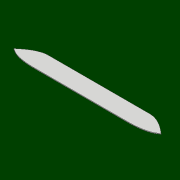
# Autodesk Inventor part: Part3
Saved by Autodesk Inventor 2018 (Build 220112000, 112)
## iProperties
Created: 2021-12-12
Part Number: Part3
Material: 一般
Document SubType Name: Modeling
Designer: gisen
Density: 1 g/cm^3
Appearance: 既定
Author: gisen
Autodesk Inventor part; units mm, degrees
ref_plane "YZ Plane" through (0, 0, 0) normal (1, 0, 0) x (0, 1, 0)
ref_plane "XZ Plane" through (0, 0, 0) normal (0, 1, 0) x (-1, 0, 0)
ref_plane "XY Plane" through (0, 0, 0) normal (0, 0, 1) x (1, 0, 0)
sketch "スケッチ1" plane through (0, 0, 0) normal (0, 0, 1) x (1, 0, 0)
  line L0 (357.9651, 235.4843) -> (362.63, 235.5738)
  line L1 (362.63, 235.5738) -> (367.0044, 235.8303)
  line L2 (367.0044, 235.8303) -> (371.0643, 236.2346)
  line L3 (371.0643, 236.2346) -> (374.8054, 236.7675)
  line L4 (374.8054, 236.7675) -> (378.2233, 237.4103)
  line L5 (378.2233, 237.4103) -> (381.3146, 238.1447)
  line L6 (381.3146, 238.1447) -> (384.0762, 238.953)
  line L7 (384.0762, 238.953) -> (386.507, 239.8191)
  line L8 (386.507, 239.8191) -> (388.6078, 240.7295)
  line L9 (388.6078, 240.7295) -> (390.3342, 241.6502)
  line L10 (390.3342, 241.6502) -> (395.2502, 244.5906)
  line L11 (395.2502, 244.5906) -> (390.8507, 248.2071)
  line L12 (390.8507, 248.2071) -> (388.6394, 249.9662)
  line L13 (388.6394, 249.9662) -> (386.4174, 251.6158)
  line L14 (386.4174, 251.6158) -> (384.2013, 253.1435)
  line L15 (384.2013, 253.1435) -> (381.995, 254.5468)
  line L16 (381.995, 254.5468) -> (379.8025, 255.8227)
  line L17 (379.8025, 255.8227) -> (377.6276, 256.9685)
  line L18 (377.6276, 256.9685) -> (375.4738, 257.9812)
  line L19 (375.4738, 257.9812) -> (373.3448, 258.8578)
  line L20 (373.3448, 258.8578) -> (371.2439, 259.5946)
  line L21 (371.2439, 259.5946) -> (369.1946, 260.1821)
  line L22 (369.1946, 260.1821) -> (368.499, 260.3499)
  line L23 (368.499, 260.3499) -> (367.8292, 260.4961)
  line L24 (367.8292, 260.4961) -> (367.1644, 260.6258)
  line L25 (367.1644, 260.6258) -> (366.5049, 260.7386)
  line L26 (366.5049, 260.7386) -> (365.8512, 260.8345)
  line L27 (365.8512, 260.8345) -> (365.2034, 260.9133)
  line L28 (365.2034, 260.9133) -> (364.5618, 260.9749)
  line L29 (364.5618, 260.9749) -> (363.9265, 261.0192)
  line L30 (363.9265, 261.0192) -> (363.298, 261.0459)
  line L31 (363.298, 261.0459) -> (362.6912, 261.0547)
  line L32 (362.6912, 261.0547) -> (216.4134, 261.0547)
  line L33 (216.4134, 261.0547) -> (215.8059, 261.0459)
  line L34 (215.8059, 261.0459) -> (215.1769, 261.0192)
  line L35 (215.1769, 261.0192) -> (214.5413, 260.9749)
  line L36 (214.5413, 260.9749) -> (213.8996, 260.9133)
  line L37 (213.8996, 260.9133) -> (213.2517, 260.8345)
  line L38 (213.2517, 260.8345) -> (212.598, 260.7385)
  line L39 (212.598, 260.7385) -> (211.9388, 260.6257)
  line L40 (211.9388, 260.6257) -> (211.2743, 260.4961)
  line L41 (211.2743, 260.4961) -> (210.6048, 260.3498)
  line L42 (210.6048, 260.3498) -> (209.9101, 260.1821)
  line L43 (209.9101, 260.1821) -> (207.861, 259.5948)
  line L44 (207.861, 259.5948) -> (205.76, 258.858)
  line L45 (205.76, 258.858) -> (203.631, 257.9815)
  line L46 (203.631, 257.9815) -> (201.4773, 256.9688)
  line L47 (201.4773, 256.9688) -> (199.3024, 255.8229)
  line L48 (199.3024, 255.8229) -> (197.1099, 254.5469)
  line L49 (197.1099, 254.5469) -> (194.9035, 253.1437)
  line L50 (194.9035, 253.1437) -> (192.6871, 251.6159)
  line L51 (192.6871, 251.6159) -> (190.4648, 249.9663)
  line L52 (190.4648, 249.9663) -> (188.253, 248.2073)
  line L53 (188.253, 248.2073) -> (183.8515, 244.5903)
  line L54 (183.8515, 244.5903) -> (188.7703, 241.6499)
  line L55 (188.7703, 241.6499) -> (190.4975, 240.7294)
  line L56 (190.4975, 240.7294) -> (192.5987, 239.8191)
  line L57 (192.5987, 239.8191) -> (195.0298, 238.953)
  line L58 (195.0298, 238.953) -> (197.7916, 238.1447)
  line L59 (197.7916, 238.1447) -> (200.8827, 237.4103)
  line L60 (200.8827, 237.4103) -> (204.3004, 236.7675)
  line L61 (204.3004, 236.7675) -> (208.0411, 236.2346)
  line L62 (208.0411, 236.2346) -> (212.1004, 235.8303)
  line L63 (212.1004, 235.8303) -> (216.4741, 235.5738)
  line L64 (216.4741, 235.5738) -> (221.1379, 235.4843)
  line L65 (221.1379, 235.4843) -> (357.9651, 235.4843)
  point P0 (0, 0)
  constraints: 132 end point
extrude "押し出し1" add sketch "スケッチ1" along normal blind 1
